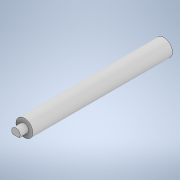
# Autodesk Inventor part: Ось 6мм задняя
Saved by Autodesk Inventor 2020 (Build 240168000, 168)
## iProperties
Created: 2021-04-13
Part Number: Ось 6мм задняя
Material: Типовые
Document SubType Name: Modeling
Designer: Антон
Density: 1 g/cm^3
Appearance: По умолчанию
Author: Антон
Autodesk Inventor part; units mm, degrees
ref_plane "YZ Plane" through (0, 0, 0) normal (1, 0, 0) x (0, 1, 0)
ref_plane "XZ Plane" through (0, 0, 0) normal (0, 1, 0) x (-1, 0, 0)
ref_plane "XY Plane" through (0, 0, 0) normal (0, 0, 1) x (1, 0, 0)
sketch "Эскиз1" plane through (0, 0, 0) normal (0, 0, 1) x (1, 0, 0)
  circle A0 centre (0, 0) radius 3
  dimension "d0" = 6
  constraints: 1 centre point, 1 coincident
  measures "d0" diameter of A0
extrude "Выдавливание1" add sketch "Эскиз1" along normal blind 52.65
sketch "Эскиз2" plane through (0, 0, 52.65) normal (0, 0, 1) x (1, 0, 0)
  circle A0 centre (0, 0) radius 1.5
  circle A1 centre (0, 0) radius 3
  line L0 (1.5, -1) -> (-1.5, -1)
  line L1 (-1.5, -1) -> (-1.5, 1)
  line L2 (-1.5, 1) -> (1.5, 1)
  line L3 (1.5, 1) -> (1.5, -1)
  line L4 (1.5, -1) -> (-1.5, 1) construction
  line L5 (-1.5, -1) -> (1.5, 1) construction
  point P0 (-1.5, 0)
  point P1 (1.118, -1)
  point P2 (-1.118, -1)
  dimension "d3" = 3
  dimension "d4" = 2
  constraints: 12 end point, 3 midpoint, 2 coincident, 2 parallel, 1 centre point, 1 horizontal, 1 perpendicular, 3 other
  measures "d4" distance of L0.end L1.end
extrude "Выдавливание2" cut sketch "Эскиз2" against normal blind 3 contours L3 L0 A0 | A0 L2 L3 | A0 L0 | A0 L1 L2 | L0 L1 A0 | A1
